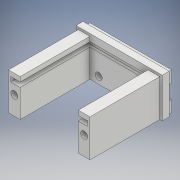
# Autodesk Inventor part: slide_sensor_clip
Saved by Autodesk Inventor 2017 (Build 210142000, 142)
## iProperties
Created: 2019-02-02
Part Number: slide_sensor_clip
Material: ABS Plastic
Document SubType Name: Modeling
Designer: simulator
Density: 1.06 g/cm^3
Appearance: Smooth - White
Mass: 2.44787 g
Surface Area: 18.1197 cm^2
Volume: 2.30931 cm^3
Author: simulator
## iProperties of the stored document slide_sensor_clip_3DPrint.ipt
Created: 2019-04-28
Part Number: slide_sensor_clip_3DPrint
Material: Generic
Document SubType Name: Modeling
Designer: simulator
Density: 1 g/cm^3
Appearance: Default
Author: simulator
Autodesk Inventor part; units mm, degrees
ref_plane "YZ Plane" through (0, 0, 0) normal (1, 0, 0) x (0, 1, 0)
ref_plane "XZ Plane" through (0, 0, 0) normal (0, 1, 0) x (-1, 0, 0)
ref_plane "XY Plane" through (0, 0, 0) normal (0, 0, 1) x (1, 0, 0)
sketch "Sketch1" plane through (0, 0, 0) normal (0, 1, 0) x (-1, 0, 0)
  line L0 (0, 0) -> (35, 0)
  line L1 (35, 0) -> (35, 6)
  line L2 (0, 6) -> (35, 6)
  line L3 (0, 0) -> (0, 6)
  line L4 (0, 6) -> (0, 0)
  line L5 (0, 3) -> (35, 3)
  line L6 (17.5, 3) -> (35, 3)
  line L7 (17.5, 3) -> (0, 3)
  point P0 (17.5, 0)
  point P1 (8.75, 3)
  point P2 (26.25, 3)
  constraints: 16 end point, 5 midpoint, 2 collinear
extrude "Extrusion1" add sketch "Sketch1" along normal blind 5
sketch "Sketch2" plane through (-35, 0, 6) normal (0, 0, 1) x (1, 0, 0)
  line L0 (0, 0) -> (35, 0) projected
  line L1 (35, 0) -> (35, 5) projected
  line L2 (0, 5) -> (35, 5) projected
  line L3 (0, 0) -> (0, 5) projected
extrude "Extrusion2" add sketch "Sketch2" along normal blind 10
sketch "Sketch3" plane through (0, 5, 0) normal (0, 1, 0) x (1, 0, 0)
  line L0 (0, 0) -> (0, -16) projected
  line L1 (0, 0) -> (-35, 0) projected
  line L2 (-35, 0) -> (-35, -16) projected
  line L3 (0, -16) -> (-35, -16) projected
  line L4 (-35, 0) -> (-35, -16) projected
  line L5 (-35, -11) -> (0, -11)
  line L6 (0, -11) -> (0, -5)
  line L7 (0, -5) -> (-35, -5)
  line L8 (-35, -5) -> (-35, -11)
  dimension "d4" = 5
  dimension "d5" = 5
  constraints: 8 end point, 2 parallel, 2 point on line, 1 horizontal, 1 perpendicular
  measures "d4" distance between parallel lines of L3 L5
  measures "d5" distance between parallel lines of L7 L1
extrude "Extrusion3" cut sketch "Sketch3" against normal blind 2 contours L0 L5 L2 L7
sketch "Sketch4" plane through (0, 0, 0) normal (0, -1, 0) x (1, 0, 0)
  line L0 (-35, 0) -> (0, 0)
  line L1 (0, 0) -> (0, 6)
  line L2 (-35, 6) -> (0, 6)
  line L3 (-35, 0) -> (-35, 6)
  line L4 (-35, 6) -> (-35, 0)
  line L5 (-35, 3) -> (0, 3)
  line L6 (-17.5, 3) -> (0, 3)
  line L7 (-17.5, 3) -> (-35, 3)
  point P0 (0, 0)
  point P1 (-17.5, 0)
  point P2 (-8.75, 3)
  point P3 (-26.25, 3)
  constraints: 16 end point, 5 midpoint, 2 collinear
hole "Hole1" at (-8.75, 0, 3) at (-26.25, 0, 3) direction (0, 1, 0) diameter 3 depth 8 tip angle 118
sketch "Sketch6" plane through (0, 0, 0) normal (0, -1, 0) x (1, 0, 0)
  circle A0 centre (-8.75, 3) radius 1.5 projected
  circle A1 centre (-26.25, 3) radius 1.5 projected
  line L0 (-35, 0) -> (-35, 16) projected
  line L1 (0, 0) -> (-35, 0) projected
  line L2 (0, 0) -> (0, 16) projected
  line L3 (-35, 16) -> (0, 16) projected
  line L4 (-35, 16) -> (-30, 16)
  line L5 (-30, 16) -> (-30, 0)
  line L6 (-30, 0) -> (-35, 0)
  line L7 (-35, 0) -> (-35, 16)
  line L8 (-35, 16) -> (0, 16) projected
  line L9 (0, 16) -> (-5, 16)
  line L10 (-5, 16) -> (-5, 0)
  line L11 (-5, 0) -> (0, 0)
  line L12 (0, 0) -> (0, 16)
  line L13 (-30, 13) -> (-5, 13)
  line L14 (-34, 14) -> (-1, 14)
  line L15 (-1, 14) -> (-1, 12)
  line L16 (-1, 12) -> (-34, 12)
  line L17 (-34, 12) -> (-34, 14)
  line L18 (-34, 14) -> (-1, 12) construction
  line L19 (-1, 14) -> (-34, 12) construction
  line L20 (-36, 17) -> (-36, 0)
  line L21 (-36, 0) -> (1, 0)
  line L22 (1, 0) -> (1, 17)
  line L23 (-36, 17) -> (1, 17)
  point P0 (-17.5, 13)
  dimension "d23" = 5
  dimension "d24" = 16
  dimension "d25" = 5
  dimension "d26" = 16
  dimension "d27" = 3
  dimension "d28" = 33
  dimension "d29" = 2
  dimension "d30" = 1
  dimension "d31" = 1
  dimension "d32" = 1
  dimension "d33" = 0
  constraints: 38 end point, 7 parallel, 4 perpendicular, 3 horizontal, 3 midpoint, 2 point on line
  measures "d23" distance of L5.end L6.end
  measures "d24" distance of L4.end L5.end
  measures "d25" distance of L11.end L10.end
  measures "d26" distance of L10.end L9.end
  measures "d27" distance between parallel lines of L3 L13
  measures "d28" distance of L15.end L16.end
  measures "d29" distance of L14.end L15.end
  measures "d30" distance between parallel lines of L23 L8
  measures "d31" distance between parallel lines of L20 L0
  measures "d32" distance between parallel lines of L2 L22
  measures "d33" distance between parallel lines of L1 L21
extrude "Extrusion5" add sketch "Sketch6" along normal blind 30 contours L0 L3 L5 L14 L17 L16 L1 | L10 L16 L15 L14 L3 L2 L1 | L16 L17 L14 L5 | L10 L14 L15 L16
extrude "Extrusion6" cut sketch "Sketch6" along normal blind 35 and the other way blind 1 contours L16 L17 L14 L5 | L5 L13 L10 L16 | L14 L10 L13 L5 | L10 L14 L15 L16
extrude "Extrusion7" add sketch "Sketch6" against normal up to surface (3 mm away) contours L21 L20 L23 L22 L2 L3 L0
sketch "Sketch7" plane through (0, -30, 0) normal (0, -1, 0) x (1, 0, 0)
  line L0 (-30, 12) -> (-34, 12) projected
  line L1 (-34, 12) -> (-34, 14) projected
  line L2 (-34, 14) -> (-30, 14) projected
  line L3 (-30, 14) -> (-30, 16) projected
  line L4 (-30, 16) -> (-35, 16) projected
  line L5 (-35, 16) -> (-35, 0) projected
  line L6 (-35, 0) -> (-30, 0) projected
  line L7 (-30, 0) -> (-30, 12) projected
  line L8 (-1, 12) -> (-5, 12) projected
  line L9 (-5, 12) -> (-5, 0) projected
  line L10 (-5, 0) -> (0, 0) projected
  line L11 (0, 0) -> (0, 16) projected
  line L12 (0, 16) -> (-5, 16) projected
  line L13 (-5, 16) -> (-5, 14) projected
  line L14 (-5, 14) -> (-1, 14) projected
  line L15 (-1, 14) -> (-1, 12) projected
  point P0 (0, 0)
sketch "Sketch8" plane through (0, -30, 0) normal (0, -1, 0) x (1, 0, 0)
  line L0 (-30, 12) -> (-34, 12) projected
  line L1 (-34, 12) -> (-34, 14) projected
  line L2 (-34, 14) -> (-30, 14) projected
  line L3 (-30, 14) -> (-30, 16) projected
  line L4 (-30, 16) -> (-35, 16) projected
  line L5 (-35, 16) -> (-35, 0) projected
  line L6 (-35, 0) -> (-30, 0) projected
  line L7 (-30, 0) -> (-30, 12) projected
  line L8 (-1, 12) -> (-5, 12) projected
  line L9 (-5, 12) -> (-5, 0) projected
  line L10 (-5, 0) -> (0, 0) projected
  line L11 (0, 0) -> (0, 16) projected
  line L12 (0, 16) -> (-5, 16) projected
  line L13 (-5, 16) -> (-5, 14) projected
  line L14 (-5, 14) -> (-1, 14) projected
  line L15 (-1, 14) -> (-1, 12) projected
  line L16 (-35, 16) -> (-30, 0)
  line L17 (-5, 0) -> (0, 16)
  point P0 (0, 0)
  point P1 (-32.5, 8)
  point P2 (-2.5, 8)
  constraints: 4 end point, 2 midpoint
hole "Hole2" at (-32.5, -30, 8) at (-2.5, -30, 8) direction (0, 1, 0) diameter 3 depth 8 tip angle 118
body "Solid1"
